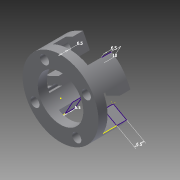
# Autodesk Inventor part: male bayonet connector - mk2
Saved by Autodesk Inventor 2015 (Build 190159000, 159)
## iProperties
Created: 2014-06-11
Part Number: male bayonet connector - mk2
Material: Generic
Document SubType Name: Modeling
Designer: ericd_000
Density: 1 g/cm^3
Appearance: Default
Author: ericd_000
Autodesk Inventor part; units mm, degrees
ref_plane "YZ Plane" through (0, 0, 0) normal (1, 0, 0) x (0, 1, 0)
ref_plane "XZ Plane" through (0, 0, 0) normal (0, 1, 0) x (-1, 0, 0)
ref_plane "XY Plane" through (0, 0, 0) normal (0, 0, 1) x (1, 0, 0)
sketch "Sketch1" plane through (0, 0, 0) normal (0, 1, 0) x (-1, 0, 0)
  circle A0 centre (0, 0) radius 25
  circle A1 centre (0, 0) radius 15
  dimension "d0" = 50
  dimension "d1" = 30
  constraints: 2 centre point, 2 coincident
  measures "d0" diameter of A0
  measures "d1" diameter of A1
extrude "Extrusion1" add sketch "Sketch1" along normal blind 6
sketch "Sketch2" plane through (0, 6, 0) normal (0, 1, 0) x (1, 0, 0)
  arc A0 (-6.6718, -13.4346) -> (-7.1782, 13.1709) centre (0, 0) ccw
  arc A1 (-21.9516, -11.9636) -> (-11.1196, -22.3909) centre (0, 0) ccw
  line L0 (-13.1709, -7.1782) -> (-21.9516, -11.9636)
  line L1 (-13.4346, 6.6718) -> (-22.3909, 11.1196)
  line L2 (-7.1782, 13.1709) -> (-11.9636, 21.9516)
  circle A2 centre (0, 0) radius 15 projected
  line L3 (6.6718, 13.4346) -> (11.1196, 22.3909)
  circle A3 centre (0, 0) radius 25 projected
  line L4 (13.1709, 7.1782) -> (21.9516, 11.9636)
  line L5 (-11.1196, -22.3909) -> (-6.6718, -13.4346)
  line L6 (7.1782, -13.1709) -> (11.9636, -21.9516)
  line L7 (13.4346, -6.6718) -> (22.3909, -11.1196)
  arc A4 (-22.3909, 11.1196) -> (-21.9516, -11.9636) centre (0, 0) ccw
  arc A5 (-11.1196, -22.3909) -> (21.9516, 11.9636) centre (0, 0) ccw
  arc A6 (-11.9636, 21.9516) -> (-22.3909, 11.1196) centre (0, 0) ccw
  arc A7 (11.1196, 22.3909) -> (-11.9636, 21.9516) centre (0, 0) ccw
  arc A8 (21.9516, 11.9636) -> (11.1196, 22.3909) centre (0, 0) ccw
  arc A9 (-13.1709, -7.1782) -> (-6.6718, -13.4346) centre (0, 0) ccw
  arc A10 (-13.4346, 6.6718) -> (-13.1709, -7.1782) centre (0, 0) ccw
  arc A11 (-7.1782, 13.1709) -> (-13.4346, 6.6718) centre (0, 0) ccw
  dimension "d6" = 35
  dimension "d7" = 35
  dimension "d8" = 35
  dimension "d9" = 35
  dimension "d10" = 55
  dimension "d11" = 55
  dimension "d12" = 55
  dimension "d13" = 55
  constraints: 59 point on circle, 24 line through centre, 16 end point, 10 centre point, 2 coincident, 16 other
  measures "d6" angle of L0 L5
  measures "d7" angle of L2 L1
  measures "d8" angle of L4 L3
  measures "d9" angle of L7 L6
  measures "d10" angle of L5 L6
  measures "d11" angle of L1 L0
  measures "d12" angle of L3 L2
  measures "d13" angle of L4 L7
extrude "Extrusion2" add sketch "Sketch2" along normal blind 15.5 contours L5 A1 L0 A2 | A0 L7 A3 L6 | L1 A3 L2 A2 | A0 L3 A3 L4
sketch "Sketch3" plane through (11.9636, 6, 21.9516) normal (-0.8781, 0, 0.4785) x (0.4785, 0, 0.8781)
  line L0 (-10, 15.5) -> (0, 15.5)
  line L1 (0, 15.5) -> (0, 9)
  line L2 (0, 9) -> (-10, 9)
  line L3 (-10, 9) -> (-10, 15.5)
  point P0 (-25, -6)
  dimension "d18" = 6.5
  dimension "d21" = 10
  constraints: 8 end point, 2 parallel, 1 horizontal, 1 perpendicular
  measures "d18" distance between parallel lines of L0 L2
  measures "d21" distance between parallel lines of L3 L1
sketch "Sketch4" plane through (-21.9516, 6, 11.9636) normal (-0.4785, 0, -0.8781) x (-0.8781, 0, 0.4785)
  line L0 (0, 0) -> (0, 15.5) projected
  line L1 (-10, 15.5) -> (0, 15.5)
  line L2 (0, 15.5) -> (0, 9)
  line L3 (0, 9) -> (-10, 9)
  line L4 (-10, 9) -> (-10, 15.5)
  point P0 (-25, -6)
  dimension "d20" = 6.5
  constraints: 8 end point, 2 parallel, 1 horizontal, 1 perpendicular, 1 point on line
  measures "d20" distance between parallel lines of L1 L3
sketch "Sketch5" plane through (-11.9636, 6, -21.9516) normal (0.8781, 0, -0.4785) x (-0.4785, 0, -0.8781)
  line L0 (0, 0) -> (0, 15.5) projected
  line L1 (-10, 15.5) -> (0, 15.5)
  line L2 (0, 15.5) -> (0, 9)
  line L3 (0, 9) -> (-10, 9)
  line L4 (-10, 9) -> (-10, 15.5)
  point P0 (-25, -6)
  dimension "d19" = 6.5
  constraints: 8 end point, 2 parallel, 1 horizontal, 1 perpendicular, 1 point on line
  measures "d19" distance between parallel lines of L1 L3
sketch "Sketch6" plane through (21.9516, 6, -11.9636) normal (0.4785, 0, 0.8781) x (0.8781, 0, -0.4785)
  point P0 (-25, -6)
sketch "Sketch7" plane through (21.9516, 6, -11.9636) normal (0.4785, 0, 0.8781) x (0.8781, 0, -0.4785)
  line L0 (0, 0) -> (0, 15.5) projected
  line L1 (-10, 15.5) -> (0, 15.5)
  line L2 (0, 15.5) -> (0, 9)
  line L3 (0, 9) -> (-10, 9)
  line L4 (-10, 9) -> (-10, 15.5)
  point P0 (-25, -6)
  dimension "d17" = 6.5
  constraints: 8 end point, 2 parallel, 1 horizontal, 1 perpendicular, 1 point on line
  measures "d17" distance between parallel lines of L3 L1
sketch "Sketch12" plane through (-6.6718, 6, 13.4346) normal (0.8956, 0, 0.4448) x (0.4448, 0, -0.8956)
  line L0 (0, 0) -> (0, 15.5) projected
  line L1 (-10, 15.5) -> (0, 15.5)
  line L2 (0, 15.5) -> (0, 8.5)
  line L3 (0, 8.5) -> (-10, 8.5)
  line L4 (-10, 8.5) -> (-10, 15.5)
  point P0 (15, -6)
  dimension "d55" = 7
  constraints: 8 end point, 2 parallel, 1 horizontal, 1 perpendicular, 1 point on line
  measures "d55" distance between parallel lines of L1 L3
sketch "Sketch13" plane through (13.4346, 6, 6.6718) normal (0.4448, 0, -0.8956) x (-0.8956, 0, -0.4448)
  line L0 (0, 0) -> (0, 15.5) projected
  line L1 (-10, 15.5) -> (0, 15.5)
  line L2 (0, 15.5) -> (0, 8.5)
  line L3 (0, 8.5) -> (-10, 8.5)
  line L4 (-10, 8.5) -> (-10, 15.5)
  point P0 (15, -6)
  dimension "d56" = 7
  constraints: 8 end point, 2 parallel, 1 horizontal, 1 perpendicular, 1 point on line
  measures "d56" distance between parallel lines of L3 L1
sketch "Sketch14" plane through (6.6718, 6, -13.4346) normal (-0.8956, 0, -0.4448) x (-0.4448, 0, 0.8956)
  line L0 (-10, 15.5) -> (0, 15.5)
  line L1 (0, 15.5) -> (0, 8.5)
  line L2 (0, 8.5) -> (-10, 8.5)
  line L3 (-10, 8.5) -> (-10, 15.5)
  point P0 (15, -6)
  dimension "d57" = 7
  constraints: 8 end point, 2 parallel, 1 horizontal, 1 perpendicular
  measures "d57" distance between parallel lines of L0 L2
sketch "Sketch15" plane through (-13.4346, 6, -6.6718) normal (-0.4448, 0, 0.8956) x (0.8956, 0, 0.4448)
  line L0 (0, 0) -> (0, 15.5) projected
  line L1 (-10, 15.5) -> (0, 15.5)
  line L2 (0, 15.5) -> (0, 8.5)
  line L3 (0, 8.5) -> (-10, 8.5)
  line L4 (-10, 8.5) -> (-10, 15.5)
  point P0 (15, -6)
  dimension "d58" = 7
  constraints: 8 end point, 2 parallel, 1 horizontal, 1 perpendicular, 1 point on line
  measures "d58" distance between parallel lines of L1 L3
extrude "Extrusion11" add sketch "Sketch12" along normal blind 5
extrude "Extrusion12" add sketch "Sketch13" along normal blind 5
sketch "Sketch16" plane through (6.6718, 6, -13.4346) normal (-0.8956, 0, -0.4448) x (-0.4448, 0, 0.8956)
  point P0 (15, -6)
extrude "Extrusion13" add sketch "Sketch14" along normal blind 5
extrude "Extrusion14" add sketch "Sketch15" along normal blind 5
sketch "Sketch8" plane through (0, 21.5, 0) normal (0, 1, 0) x (1, 0, 0)
  circle A0 centre (-16.8241, 10.5881) radius 3
  arc A1 (-7.1782, 13.1709) -> (-13.4346, 6.6718) centre (0, 0) ccw projected
  line L0 (-7.5733, 24.3443) -> (-2.7879, 15.5637) projected
  arc A2 (-11.9636, 21.9516) -> (-22.3909, 11.1196) centre (0, 0) ccw projected
  circle A3 centre (0, 0) radius 25 projected
  line L1 (-22.3909, 11.1196) -> (-13.4346, 6.6718) projected
  line L2 (-15.6585, 2.1936) -> (-24.6149, 6.6414) projected
  line L3 (-16.8241, 10.5881) -> (-12.6951, 7.9896) construction
  dimension "d30" = 6
  dimension "d71" = 7
  dimension "d72" = 4.129
  constraints: 2 end point, 1 centre point, 1 line through centre, 1 point on circle
  measures "d30" diameter of A0
  measures "d71" distance from line of L2 L3.start
  measures "d72" horizontal distance of L3.start L3.end
sketch "Sketch9" plane through (0, 21.5, 0) normal (0, 1, 0) x (1, 0, 0)
  circle A0 centre (10.6983, 17.046) radius 3
  line L0 (24.3443, 7.5733) -> (15.5637, 2.7879) construction
  arc A1 (21.9516, 11.9636) -> (11.1196, 22.3909) centre (0, 0) ccw construction
  line L1 (11.1196, 22.3909) -> (6.6718, 13.4346) projected
  line L2 (2.1936, 15.6585) -> (6.6414, 24.6149) projected
  line L3 (10.6983, 17.046) -> (13.2898, 21.175) construction
  dimension "d37" = 6
  dimension "d73" = 7
  dimension "d77" = 4.129
  constraints: 2 end point, 1 centre point, 1 line through centre, 1 point on circle
  measures "d37" diameter of A0
  measures "d73" distance from line of L2 L3.start
  measures "d77" vertical distance of L3.start L3.end
sketch "Sketch10" plane through (0, 21.5, 0) normal (0, 1, 0) x (1, 0, 0)
  circle A0 centre (17.046, -10.6983) radius 3
  line L0 (7.5733, -24.3443) -> (2.7879, -15.5637) projected
  arc A1 (11.9636, -21.9516) -> (22.3909, -11.1196) centre (0, 0) ccw construction
  line L1 (22.3909, -11.1196) -> (13.4346, -6.6718) projected
  line L2 (15.6585, -2.1936) -> (24.6149, -6.6414) projected
  line L3 (17.046, -10.6983) -> (21.175, -13.2898) construction
  dimension "d42" = 6
  dimension "d78" = 7
  dimension "d79" = 4.129
  constraints: 2 end point, 1 centre point, 1 line through centre, 1 point on circle
  measures "d42" diameter of A0
  measures "d78" distance from line of L2 L3.start
  measures "d79" horizontal distance of L3.start L3.end
sketch "Sketch11" plane through (0, 21.5, 0) normal (0, 1, 0) x (1, 0, 0)
  circle A0 centre (-10.5881, -16.8241) radius 3
  line L0 (-24.3443, -7.5733) -> (-15.5637, -2.7879) projected
  arc A1 (-13.1709, -7.1782) -> (-6.6718, -13.4346) centre (0, 0) ccw construction
  line L1 (-11.1196, -22.3909) -> (-6.6718, -13.4346) projected
  line L2 (-2.1936, -15.6585) -> (-6.6414, -24.6149) projected
  line L3 (-10.5881, -16.8241) -> (-7.9896, -12.6951) construction
  dimension "d44" = 6
  dimension "d80" = 7
  dimension "d83" = 4.129
  constraints: 2 end point, 1 centre point, 1 line through centre, 1 point on circle
  measures "d44" diameter of A0
  measures "d80" distance from line of L2 L3.start
  measures "d83" vertical distance of L3.start L3.end
extrude "Extrusion15" cut sketch "Sketch8" against normal through all contours A0 L1 | L1 A0
extrude "Extrusion16" cut sketch "Sketch9" against normal through all
extrude "Extrusion17" cut sketch "Sketch10" against normal through all
extrude "Extrusion18" cut sketch "Sketch11" against normal through all
sketch "Sketch17" plane through (0, 21.5, 0) normal (0, 1, 0) x (1, 0, 0)
  line L0 (2.1936, 15.6585) -> (6.6414, 24.6149) projected
  line L1 (6.6718, 13.4346) -> (2.1936, 15.6585)
  line L2 (2.1936, 15.6585) -> (4.4175, 20.1367)
  line L3 (6.6718, 13.4346) -> (5.4119, 22.139)
  point P0 (0, 0)
  constraints: 6 end point, 1 collinear, 1 midpoint, 1 perpendicular, 1 point on line
extrude "Extrusion19" cut sketch "Sketch17" against normal blind 8
body "Solid1"
